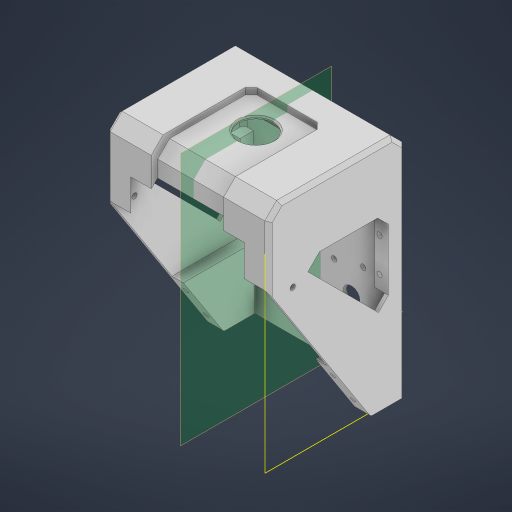
# Autodesk Inventor part: Head_base_mount
Saved by Autodesk Inventor 2024 (Build 280153000, 153)
## iProperties
Created: 2025-09-25
Part Number: Head_base_mount
Material: Generic
Document SubType Name: Modeling
Designer: kevin
Density: 1 g/cm^3
Appearance: Default
Author: kevin
Autodesk Inventor part; units mm, degrees
sketch "Sketch1" plane through (0, 0, 0) normal (0, 0, 1) x (1, 0, 0)
  circle A0 centre (57.1655, 18.417) radius 2.1 projected
  circle A1 centre (12.7885, 12.5269) radius 2.1 projected
  circle A2 centre (17.2869, -26.8107) radius 2.1 projected
  circle A3 centre (-1.1004, -6.0436) radius 5 projected
  line L0 (64.4194, 6.1067) -> (62.3371, -1.6056) projected
  line L1 (67.3095, 9.3686) -> (64.4194, 6.1067) projected
  ellipse E0 centre (57.1655, 18.417) end of major axis (47.0979, 27.5508) minor radius 11.51 (67.3095, 9.3686) -> (68.6853, 21.7358) ccw projected
  ellipse E1 centre (54.4602, 15.4351) end of major axis (43.6731, 3.5452) minor radius 13.5934 (68.6853, 21.7358) -> (59.3507, 30.2045) ccw projected
  ellipse E2 centre (57.1655, 18.417) end of major axis (47.0979, 27.5508) minor radius 11.51 (59.3507, 30.2045) -> (47.0214, 27.4655) ccw projected
  line L2 (36.5043, 15.5956) -> (47.0214, 27.4655) projected
  arc A4 (36.5043, 15.5956) -> (29.6862, 12.4398) centre (33.7853, 12.5269) ccw projected
  line L3 (16.8875, 12.4398) -> (29.6862, 12.4398) projected
  arc A5 (16.8875, 12.4398) -> (10.0695, 15.5956) centre (12.7885, 12.5269) ccw projected
  line L4 (10.0695, 15.5956) -> (-0.4476, 27.4655) projected
  ellipse E3 centre (-10.5917, 18.417) end of major axis (-0.5241, 27.5508) minor radius 11.51 (-0.4476, 27.4655) -> (-12.7769, 30.2045) ccw projected
  ellipse E4 centre (-7.8864, 15.4351) end of major axis (2.9006, 3.5452) minor radius 13.5934 (-12.7769, 30.2045) -> (-22.1115, 21.7358) ccw projected
  ellipse E5 centre (-10.5917, 18.417) end of major axis (-0.5241, 27.5508) minor radius 11.51 (-22.1115, 21.7358) -> (-20.7358, 9.3686) ccw projected
  line L5 (-20.7358, 9.3686) -> (-17.8456, 6.1067) projected
  line L6 (-17.8456, 6.1067) -> (-15.7633, -1.6056) projected
  line L7 (-15.7633, -1.6056) -> (-6.4546, -11.2249) projected
  line L8 (-6.4546, -11.2249) -> (1.9738, -21.6241) projected
  line L9 (1.9738, -21.6241) -> (9.6038, -24.7107) projected
  line L10 (9.6038, -24.7107) -> (14.4693, -29.7892) projected
  arc A6 (14.4693, -29.7892) -> (17.2869, -30.9107) centre (17.2869, -26.8107) ccw projected
  line L11 (17.2869, -30.9107) -> (29.2869, -30.9107) projected
  arc A7 (29.2869, -30.9107) -> (32.1045, -29.7892) centre (29.2869, -26.8107) ccw projected
  line L12 (36.97, -24.7107) -> (32.1045, -29.7892) projected
  line L13 (44.6, -21.6241) -> (36.97, -24.7107) projected
  line L14 (53.0284, -11.2249) -> (44.6, -21.6241) projected
  line L15 (62.3371, -1.6056) -> (53.0284, -11.2249) projected
  circle A8 centre (-10.5917, 18.417) radius 2.1 projected
  circle A9 centre (47.6742, -6.0436) radius 5 projected
  circle A10 centre (29.2869, -26.8107) radius 2.1 projected
  circle A11 centre (33.7853, 12.5269) radius 2.1 projected
  line L16 (23.0369, -57.3492) -> (23.0369, -47.5992) projected
  line L17 (88.0369, 125.5308) -> (-41.9631, 125.5308)
  line L18 (-41.9631, 125.5308) -> (-41.9631, -57.3492)
  line L19 (-41.9631, -57.3492) -> (88.0369, -57.3492)
  line L20 (88.0369, -57.3492) -> (88.0369, 125.5308)
  line L21 (88.0369, 125.5308) -> (-41.9631, -57.3492) construction
  line L22 (-41.9631, 125.5308) -> (88.0369, -57.3492) construction
  circle A12 centre (47.6742, -6.0436) radius 6.75
  circle A13 centre (-1.1004, -6.0436) radius 6.75
  line L23 (33.1369, 106.1308) -> (33.1369, 113.8808) projected
  line L24 (12.9369, 113.8808) -> (12.9369, 106.1308) projected
  line L25 (33.1369, 110.0058) -> (12.9369, 110.0058) construction
  circle A14 centre (34.0369, 59.4461) radius 2.1
  circle A15 centre (23.0369, 69.6441) radius 2.1
  circle A16 centre (12.0369, 59.4461) radius 2.1
  line L26 (23.0369, 12.4398) -> (23.0369, -30.9107) construction
  arc A17 (10.7829, 39.5316) -> (35.2909, 39.5316) centre (23.0369, 31.7099) ccw construction
  line L27 (23.0369, 31.7099) -> (23.0369, -30.9107) construction
  line L28 (23.0369, 31.7099) -> (23.0369, 44.0027) construction
  point P0 (0, 0)
  point P1 (23.0369, 34.0908)
  dimension "d0" = 130
  dimension "d1" = 182.88
  dimension "d2" = 1.75
  dimension "d3" = 1.75
  dimension "d49" = 4.2
  dimension "d51" = 4.2
  dimension "d52" = 15
  constraints: 20 end point, 6 centre point, 4 midpoint, 3 parallel, 2 point on circle, 2 point on line, 2 vertical, 1 horizontal, 1 perpendicular, 10 other
  measures "d0" distance of L19.end L18.end
  measures "d1" distance of L18.end L17.end
  measures "d2" radial gap between concentric circles of A9 A12
  measures "d3" radial gap between concentric circles of A3 A13
  measures "d49" diameter of A14
  measures "d51" diameter of A15
  measures "d52" distance of A15.centre A14.centre
extrude "Extrusion1" add sketch "Sketch1" along normal blind 3 contours L0 L15 L14 L13 L12 A7 L11 A6 L10 L9 L8 L7 L6 L5 E5 E4 E3 L4 A5 L3 A4 L2 E2 E1 E0 L1 | L20 L19 L18 L17
ref_plane "Work Plane1" through (0, 0, 55) normal (0, 0, -1) x (-1, 0, 0)
ref_plane "Work Plane2" through (23.0369, -57.3492, 0) normal (-1, 0, 0) x (0, 0, 1)
ref_plane "Work Plane3" through (-41.9631, 120.0308, 0) normal (0, 1, 0) x (1, 0, 0)
ref_plane "Work Plane5" through (85.0369, 95.5308, 39.1468) normal (0, 0, -1) x (-1, 0, 0)
sketch "Sketch3" plane through (85.0369, 95.5308, 39.1468) normal (0, 0, -1) x (-1, 0, 0)
  line L0 (51.9, 10.6) -> (51.9, 18.35) projected
  line L1 (51.9, 18.35) -> (72.1, 18.35) projected
  line L2 (72.1, 18.35) -> (72.1, 10.6) projected
  line L3 (72.1, 10.6) -> (51.9, 10.6) projected
  line L4 (108.35, 2) -> (15.65, 2) projected
  line L5 (108.35, 22.6942) -> (108.35, 2) projected
  line L6 (87.7096, 24.5) -> (108.35, 22.6942) projected
  line L7 (36.2904, 24.5) -> (87.7096, 24.5) projected
  line L8 (15.65, 22.6942) -> (36.2904, 24.5) projected
  line L9 (15.65, 22.6942) -> (15.65, 2) projected
  line L10 (72.5, 18.75) -> (51.5, 18.75)
  line L11 (51.5, 18.75) -> (51.5, 10.2)
  line L12 (51.5, 10.2) -> (72.5, 10.2)
  line L13 (72.5, 10.2) -> (72.5, 18.75)
  line L14 (51.5, 18.35) -> (39.8, 18.35)
  line L15 (39.8, 18.35) -> (39.8, 10.6)
  line L16 (39.8, 10.6) -> (51.5, 10.6)
  line L17 (62, 18.35) -> (62, 14.8844) construction
  line L18 (39.8, 18.35) -> (15.65, 18.75)
  line L19 (39.8, 10.6) -> (15.65, 11)
  line L20 (72.5, 18.35) -> (84.2, 18.35)
  line L21 (84.2, 18.35) -> (84.2, 10.6)
  line L22 (84.2, 10.6) -> (72.5, 10.6)
  line L23 (84.2, 18.35) -> (108.35, 18.75)
  line L24 (84.2, 10.6) -> (108.35, 11)
  point P0 (85.0369, -95.5308)
  point P1 (108.35, 11)
  point P2 (108.35, 18.75)
  dimension "d8" = 0.4
  dimension "d9" = 11.7
  constraints: 30 end point, 6 symmetric about line, 4 point on line, 2 perpendicular, 1 horizontal, 1 midpoint, 1 parallel, 1 vertical, 3 other
  measures "d8" distance between parallel lines of L1 L10
  measures "d9" distance of L14.start L14.end
extrude "Extrusion2" add sketch "Sketch3" along normal blind 9.398 contours L4 L9 L19 L16 L11 L12 L13 L22 L24 L5 | L23 L20 L13 L10 L11 L14 L18 L9 L8 L7 L6 L5 | L22 L13 L20 L21 | L15 L14 L11 L16
sketch "Sketch4" plane through (0.8369, 106.1308, 39.1468) normal (-1, 0, 0) x (0, 0, 1)
  circle A0 centre (-4.6468, 3.875) radius 2.25 projected
  point P0 (-39.1468, -106.1308)
extrude "Extrusion3" cut sketch "Sketch4" against normal up to surface (44.4 mm away)
sketch "Sketch5" plane through (0.8369, 106.1308, 39.1468) normal (-1, 0, 0) x (0, 0, 1)
  circle A0 centre (-4.6468, 3.875) radius 2.25 projected
  circle A1 centre (-4.6468, 3.875) radius 3.3
  point P0 (-39.1468, -106.1308)
  dimension "d14" = 6.6
  constraints: 1 centre point, 1 coincident
  measures "d14" diameter of A1
extrude "Extrusion4" cut sketch "Sketch5" against normal blind 3.5
sketch "Sketch6" plane through (45.2369, 106.1308, 39.1468) normal (1, 0, 0) x (0, 0, -1)
  circle A0 centre (4.6468, 3.875) radius 2.25 projected
  circle A1 centre (4.6468, 3.875) radius 3.3
  point P0 (39.1468, -106.1308)
  dimension "d17" = 6.6
  constraints: 1 centre point, 1 coincident
  measures "d17" diameter of A1
extrude "Extrusion5" cut sketch "Sketch6" against normal blind 3.5 contours A0 | A1
sketch "Sketch7" plane through (85.0369, 95.5308, 29.7488) normal (0, 0, -1) x (-1, 0, 0)
  line L0 (15.65, 11) -> (15.65, 2) projected
  line L1 (15.65, 2) -> (108.35, 2) projected
  line L2 (108.35, 2) -> (108.35, 11) projected
  line L3 (108.35, 11) -> (84.2, 10.6) projected
  line L4 (84.2, 10.6) -> (84.2, 18.35) projected
  line L5 (84.2, 18.35) -> (108.35, 18.75) projected
  line L6 (108.35, 18.75) -> (108.35, 22.6942) projected
  line L7 (108.35, 22.6942) -> (87.7096, 24.5) projected
  line L8 (87.7096, 24.5) -> (36.2904, 24.5) projected
  line L9 (36.2904, 24.5) -> (15.65, 22.6942) projected
  line L10 (15.65, 22.6942) -> (15.65, 18.75) projected
  line L11 (15.65, 18.75) -> (39.8, 18.35) projected
  line L12 (39.8, 18.35) -> (39.8, 10.6) projected
  line L13 (39.8, 10.6) -> (15.65, 11) projected
  line L14 (51.5, 10.2) -> (51.5, 18.75) projected
  line L15 (51.5, 18.75) -> (72.5, 18.75) projected
  line L16 (72.5, 18.75) -> (72.5, 10.2) projected
  line L17 (72.5, 10.2) -> (51.5, 10.2) projected
  line L18 (15.65, 11) -> (15.65, 18.75)
  line L19 (108.35, 18.75) -> (108.35, 11)
  point P0 (85.0369, -95.5308)
  constraints: 4 end point, 1 parallel, 1 point on line
extrude "Extrusion6" add sketch "Sketch7" along normal up to surface (26.7488 mm away) contours L13 L12 L11 L10 L9 L8 L7 L6 L5 L4 L3 L2 L1 L0 | L18 L11 L12 L13 | L3 L4 L5 L19 | L14 L15 L16 L17
sketch "Sketch8" plane through (0, 0, 3) normal (0, 0, 1) x (1, 0, 0)
  line L0 (69.3869, 97.5308) -> (-23.3131, 97.5308) projected
  line L1 (-23.3131, 97.5308) -> (-23.3131, 118.225) projected
  line L2 (-23.3131, 118.225) -> (-2.6727, 120.0308) projected
  line L3 (-2.6727, 120.0308) -> (48.7465, 120.0308) projected
  line L4 (48.7465, 120.0308) -> (69.3869, 118.225) projected
  line L5 (69.3869, 118.225) -> (69.3869, 97.5308) projected
  line L6 (-41.9631, -57.3492) -> (88.0369, -57.3492) projected
  line L7 (88.0369, -57.3492) -> (88.0369, 125.5308) projected
  line L8 (88.0369, 125.5308) -> (-41.9631, 125.5308) projected
  line L9 (-41.9631, 125.5308) -> (-41.9631, -57.3492) projected
  circle A0 centre (12.7885, 12.5269) radius 2.1 projected
  circle A1 centre (33.7853, 12.5269) radius 2.1 projected
  circle A2 centre (47.6742, -6.0436) radius 6.75 projected
  circle A3 centre (-1.1004, -6.0436) radius 6.75 projected
  circle A4 centre (29.2869, -26.8107) radius 2.1 projected
  circle A5 centre (-10.5917, 18.417) radius 2.1 projected
  circle A6 centre (17.2869, -26.8107) radius 2.1 projected
  circle A7 centre (57.1655, 18.417) radius 2.1 projected
  line L10 (85.0369, 122.5308) -> (85.0369, -57.3492)
  line L11 (85.0369, -54.3492) -> (-38.9631, -54.3492) construction
  line L12 (-38.9631, -57.3492) -> (-38.9631, 122.5308)
  line L13 (-38.9631, 122.5308) -> (85.0369, 122.5308) construction
  line L14 (-23.3131, 114.2808) -> (-38.9631, 114.2808)
  line L15 (23.0369, -93.9252) -> (23.0369, 162.1068) construction
  line L16 (69.3869, 114.2808) -> (85.0369, 114.2808)
  line L17 (85.0369, -52.3492) -> (-38.9631, -52.3492) construction
  point P0 (0, 0)
  dimension "d23" = 3
  dimension "d24" = 2
  constraints: 14 end point, 5 point on line, 2 symmetric about line, 1 parallel, 1 perpendicular
  measures "d23" distance between parallel lines of L7 L10
  measures "d24" distance between parallel lines of L11 L17
extrude "Extrusion7" add sketch "Sketch8" along normal blind 27 contours L5 L4 L3 L2 L1 L14 L12 L6 L9 L8 L7 L10 L16
sketch "Sketch9" plane through (0, 0, 30) normal (0, 0, 1) x (1, 0, 0)
  line L0 (69.3869, 114.2808) -> (69.3869, 118.225) projected
  line L1 (69.3869, 114.2808) -> (85.0369, 114.2808) projected
  line L2 (85.0369, 114.2808) -> (85.0369, -57.3492) projected
  line L3 (85.0369, -57.3492) -> (88.0369, -57.3492) projected
  line L4 (88.0369, -57.3492) -> (88.0369, 125.5308) projected
  line L5 (88.0369, 125.5308) -> (-41.9631, 125.5308) projected
  line L6 (-41.9631, 125.5308) -> (-41.9631, -57.3492) projected
  line L7 (-41.9631, -57.3492) -> (-38.9631, -57.3492) projected
  line L8 (-38.9631, -57.3492) -> (-38.9631, 114.2808) projected
  line L9 (-38.9631, 114.2808) -> (-23.3131, 114.2808) projected
  line L10 (-23.3131, 118.225) -> (-23.3131, 114.2808) projected
  line L11 (-2.6727, 120.0308) -> (-23.3131, 118.225) projected
  line L12 (48.7465, 120.0308) -> (-2.6727, 120.0308) projected
  line L13 (69.3869, 118.225) -> (48.7465, 120.0308) projected
  line L14 (-2.6945, 120.5308) -> (-23.8131, 118.6832) construction
  line L15 (-39.4631, -56.8492) -> (-41.4631, -56.8492)
  line L16 (87.5369, -56.8492) -> (85.5369, -56.8492)
  line L17 (69.8869, 118.6832) -> (48.7683, 120.5308) construction
  line L18 (52.0369, 120.5308) -> (-5.9631, 120.5308)
  line L19 (-2.7818, 122.5308) -> (52.0369, 122.5308)
  line L20 (88.0369, 125.5308) -> (-41.9631, 125.5308) projected
  line L21 (52.0369, 125.5308) -> (52.0369, 106.9413)
  line L22 (58.0369, 122.5308) -> (-5.9631, 122.5308)
  line L23 (23.0369, 125.5308) -> (23.0369, 133.2517) construction
  line L24 (-5.9631, 125.5308) -> (-5.9631, 106.9413)
  line L25 (88.0369, 120.5308) -> (52.0369, 120.5308)
  line L26 (-5.9631, 120.5308) -> (-41.9631, 120.5308)
  line L27 (-41.9631, 116.0058) -> (-41.9631, 125.5308) projected
  line L28 (-38.9631, 114.2808) -> (-38.9631, 120.5308)
  line L29 (85.0369, 114.2808) -> (85.0369, 120.5308)
  point P0 (0, 0)
  point P1 (52.0369, 120.2449)
  point P2 (26.13, 122.5308)
  point P3 (-5.9631, 125.5308)
  dimension "d30" = 0.5
  dimension "d31" = 2
  dimension "d32" = 36
  dimension "d38" = 5
  dimension "d40" = 5
  constraints: 28 end point, 13 point on line, 4 perpendicular, 2 symmetric about line, 2 vertical, 1 midpoint
  measures "d30" distance between parallel lines of L12 L18
  measures "d31" distance between parallel lines of L18 L19
  measures "d32" distance between parallel lines of L4 L21
  measures "d38" distance between parallel lines of L5 L25
  measures "d40" distance between parallel lines of L5 L26
ref_plane "Work Plane6" through (23.0369, 120.0308, 55) normal (0, 1, 0) x (-1, 0, 0)
sketch "Sketch10" plane through (23.0369, 120.0308, 55) normal (0, 1, 0) x (-1, 0, 0)
  circle A0 centre (0, 0) radius 11.975 projected
  circle A1 centre (0, 0) radius 7.8185 projected
  circle A2 centre (0, 0) radius 13.975
  point P0 (23.0369, -55)
  dimension "d33" = 2
  constraints: 1 centre point
  measures "d33" radial gap between concentric circles of A0 A2
extrude "Extrusion8" add sketch "Sketch9" along normal blind 80 contours L29 L25 L4 L3 L2 | L25 L21 L5 L4 | L18 L24 L22 L19 L21 | L26 L6 L5 L24 | L28 L8 L7 L6 L26
extrude "Extrusion9" cut sketch "Sketch10" along normal blind 80 contours A0 | A1 | A2
sketch "Sketch11" plane through (-41.9631, 125.5308, 0) normal (0, 1, 0) x (1, 0, 0)
  line L0 (130, 0) -> (0, 0) projected
  line L1 (0, 0) -> (0, -110) projected
  line L2 (36, -110) -> (0, -110) projected
  line L3 (36, -30) -> (36, -110) projected
  line L4 (94, -30) -> (36, -30) projected
  line L5 (94, -30) -> (94, -110) projected
  line L6 (130, -110) -> (94, -110) projected
  line L7 (130, 0) -> (130, -110) projected
  point P0 (41.9631, 0)
extrude "Extrusion10" add sketch "Sketch11" along normal blind 2
sketch "Sketch12" plane through (85.0369, -57.3492, 3) normal (-1, 0, 0) x (0, 0, 1)
  line L0 (0, 0) -> (0, 171.63) projected
  line L1 (0, 0) -> (107, 0) projected
  line L2 (107, 177.88) -> (107, 0) projected
  line L3 (27, 177.88) -> (107, 177.88) projected
  line L4 (27, 171.63) -> (27, 177.88) projected
  line L5 (0, 171.63) -> (27, 171.63) projected
  line L6 (107, 152.1906) -> (81.3106, 177.88)
  line L7 (67.65, 175.5742) -> (67.65, 154.88) construction
  point P0 (-3, 57.3492)
  dimension "d43" = 45
  constraints: 2 end point, 2 point on line
  measures "d43" angle of L2 L6
extrude "Extrusion11" add sketch "Sketch12" along normal up to surface (124 mm away) contours L6 L3 L2
sketch "Sketch13" plane through (0, 0, 110) normal (0, 0, 1) x (1, 0, 0)
  line L0 (85.0369, 94.8414) -> (-38.9631, 94.8414) projected
  line L1 (85.0369, 94.8414) -> (85.0369, -57.3492) projected
  line L2 (85.0369, -57.3492) -> (88.0369, -57.3492) projected
  line L3 (88.0369, -57.3492) -> (88.0369, 127.5308) projected
  line L4 (52.0369, 127.5308) -> (88.0369, 127.5308) projected
  line L5 (52.0369, 122.5308) -> (52.0369, 127.5308) projected
  line L6 (52.0369, 122.5308) -> (-5.9631, 122.5308) projected
  line L7 (-5.9631, 122.5308) -> (-5.9631, 127.5308) projected
  line L8 (-41.9631, 127.5308) -> (-5.9631, 127.5308) projected
  line L9 (-41.9631, -57.3492) -> (-41.9631, 127.5308) projected
  line L10 (-41.9631, -57.3492) -> (-38.9631, -57.3492) projected
  line L11 (-38.9631, -57.3492) -> (-38.9631, 94.8414) projected
  line L12 (52.0369, 128.7536) -> (52.0369, 94.8414)
  line L13 (-5.9631, 127.5308) -> (-5.9631, 94.8414)
  point P0 (0, 0)
  constraints: 4 end point, 2 perpendicular, 2 point on line
extrude "Extrusion12" cut sketch "Sketch13" against normal blind 5 contours L0 L13 L6 L12
fillet "Fillet2" radius 1 3 edges at (14.317, 122.5308, 65.9208) (14.317, 122.5308, 44.0792) (37.0119, 122.5308, 55) inverted yes
sketch "Sketch14" plane through (85.0369, -57.3492, 3) normal (-1, 0, 0) x (0, 0, 1)
  line L0 (107, 152.1906) -> (81.3106, 177.88) projected
  line L1 (27, 177.88) -> (81.3106, 177.88) projected
  line L2 (27, 171.63) -> (27, 177.88) projected
  line L3 (0, 171.63) -> (27, 171.63) projected
  line L4 (0, 0) -> (0, 171.63) projected
  line L5 (0, 0) -> (107, 0) projected
  line L6 (107, 152.1906) -> (107, 0) projected
  point P0 (-3, 57.3492)
sketch "Sketch15" plane through (85.0369, -57.3492, 3) normal (-1, 0, 0) x (0, 0, 1)
  line L0 (107, 152.1906) -> (81.3106, 177.88) projected
  line L1 (27, 177.88) -> (81.3106, 177.88) projected
  line L2 (27, 171.63) -> (27, 177.88) projected
  line L3 (0, 171.63) -> (27, 171.63) projected
  line L4 (0, 0) -> (0, 171.63) projected
  line L5 (0, 0) -> (107, 0) projected
  line L6 (107, 152.1906) -> (107, 0) projected
  line L7 (25, 0) -> (107, 127)
  point P0 (-3, 57.3492)
  dimension "d56" = 25
  dimension "d57" = 127
  constraints: 2 end point, 2 point on line
  measures "d56" distance of L4.start L7.start
  measures "d57" distance of L5.end L7.end
extrude "Extrusion13" cut sketch "Sketch15" along normal blind 225.25 and the other way blind 7.8486 contours L6 L5 L7
ref_plane "Work Plane7" through (54.0369, 69.6508, 110) normal (0, -1, 0) x (1, 0, 0)
sketch "Sketch19" plane through (85.0369, 95.5308, 39.1468) normal (0, 0, 1) x (1, 0, 0)
  line L0 (-51.9, 10.6) -> (-51.9, 18.35) projected
  line L1 (-51.9, 18.35) -> (-72.1, 18.35) projected
  line L2 (-72.1, 18.35) -> (-72.1, 10.6) projected
  line L3 (-72.1, 10.6) -> (-51.9, 10.6) projected
  line L4 (-108.35, 2) -> (-15.65, 2) projected
  line L5 (-108.35, 22.6942) -> (-108.35, 2) projected
  line L6 (-87.7096, 24.5) -> (-108.35, 22.6942) projected
  line L7 (-36.2904, 24.5) -> (-87.7096, 24.5) projected
  line L8 (-15.65, 22.6942) -> (-36.2904, 24.5) projected
  line L9 (-15.65, 22.6942) -> (-15.65, 2) projected
  line L10 (-108.55, 1.8) -> (-15.45, 1.8)
  line L11 (-15.45, 1.8) -> (-15.45, 22.8775)
  line L12 (-15.45, 22.8775) -> (-36.2817, 24.7)
  line L13 (-36.2817, 24.7) -> (-87.7183, 24.7)
  line L14 (-87.7183, 24.7) -> (-108.55, 22.8775)
  line L15 (-108.55, 22.8775) -> (-108.55, 1.8)
  point P0 (-85.0369, -95.5308)
  dimension "d71" = 0.2
  constraints: 12 end point, 5 other
  measures "d71" distance between parallel lines of L5 L15
extrude "Extrusion16" cut sketch "Sketch19" against normal blind 19.498 contours L3 L2 L1 L0 | L5 L6 L7 L8 L9 L4 | L15 L14 L13 L12 L11 L10
ref_plane "Work Plane9" through (23.0369, -57.3492, 0) normal (-1, 0, 0) x (0, 0, 1)
sketch "Sketch21" plane through (0, 0, 0) normal (0, 0, -1) x (-1, 0, 0)
  line L0 (23.3131, 114.2808) -> (23.5131, 114.2808) projected
  line L1 (23.3131, 97.5308) -> (23.3131, 114.2808) projected
  line L2 (-69.3869, 97.5308) -> (23.3131, 97.5308) projected
  line L3 (-69.3869, 114.2808) -> (-69.3869, 97.5308) projected
  line L4 (-69.5869, 114.2808) -> (-69.3869, 114.2808) projected
  line L5 (-69.5869, 118.4083) -> (-69.5869, 114.2808) projected
  line L6 (-48.7552, 120.2308) -> (-69.5869, 118.4083) projected
  line L7 (2.6814, 120.2308) -> (-48.7552, 120.2308) projected
  line L8 (23.5131, 118.4083) -> (2.6814, 120.2308) projected
  line L9 (23.5131, 114.2808) -> (23.5131, 118.4083) projected
  circle A0 centre (11.3131, 107.8779) radius 2.1 projected
  circle A1 centre (-23.3827, 107.8779) radius 2.1 projected
  circle A2 centre (-58.0785, 107.8779) radius 2.1 projected
  point P0 (0, 0)
ref_plane "Work Plane10" through (-23.3131, 97.5308, 19.6488) normal (0, 0, -1) x (0, 1, 0)
extrude "Extrusion17" cut sketch "Sketch21" against normal up to surface (19.6488 mm away) contours A0 | A1 | A2
sketch "Sketch22" plane through (0, 0, 0) normal (0, 0, -1) x (-1, 0, 0)
  circle A0 centre (-58.0785, 107.8779) radius 2.1 projected
  circle A1 centre (11.3131, 107.8779) radius 2.1 projected
  circle A2 centre (-23.3827, 107.8779) radius 2.1 projected
  line L0 (-88.0369, -57.3492) -> (-88.0369, 127.5308) projected
  line L1 (41.9631, -57.3492) -> (-88.0369, -57.3492) projected
  line L2 (41.9631, -57.3492) -> (41.9631, 127.5308) projected
  circle A3 centre (-23.0369, 69.6441) radius 2.1 projected
  circle A4 centre (-34.0369, 59.4461) radius 2.1 projected
  circle A5 centre (-12.0369, 59.4461) radius 2.1 projected
  circle A6 centre (-29.2869, -26.8107) radius 2.1 projected
  circle A7 centre (10.5917, 18.417) radius 2.1 projected
  circle A8 centre (-17.2869, -26.8107) radius 2.1 projected
  circle A9 centre (-57.1655, 18.417) radius 2.1 projected
  circle A10 centre (1.1004, -6.0436) radius 6.75 projected
  circle A11 centre (-47.6742, -6.0436) radius 6.75 projected
  circle A12 centre (-33.7853, 12.5269) radius 2.1 projected
  circle A13 centre (-12.7885, 12.5269) radius 2.1 projected
  circle A14 centre (11.3131, 107.8779) radius 4
  circle A15 centre (-23.3827, 107.8779) radius 4
  circle A16 centre (-58.0785, 107.8779) radius 4
  line L3 (-88.0369, 127.5308) -> (41.9631, 127.5308) projected
  point P0 (0, 0)
  dimension "d76" = 8
  dimension "d77" = 8
  dimension "d78" = 8
  constraints: 3 centre point, 3 coincident
  measures "d76" diameter of A14
  measures "d77" diameter of A15
  measures "d78" diameter of A16
extrude "Extrusion18" cut sketch "Sketch22" against normal blind 3 contours A14 | A15 | A16
chamfer "Chamfer3" distance 9.525 angle 45 4 edges at (23.0369, 127.5308, 0) (-23.9631, 127.5308, 110) (23.0369, 122.5308, 105) (70.0369, 127.5308, 110)
sketch "Sketch23" plane through (-41.9631, 127.5308, 0) normal (0, 1, 0) x (1, 0, 0)
  line L0 (130, -100.475) -> (94, -100.475) projected
  line L1 (130, -100.475) -> (130, -9.525) projected
  line L2 (0, -9.525) -> (130, -9.525) projected
  line L3 (0, -9.525) -> (0, -100.475) projected
  line L4 (36, -100.475) -> (0, -100.475) projected
  line L5 (36, -100.475) -> (36, -30) projected
  line L6 (36, -30) -> (94, -30) projected
  line L7 (94, -30) -> (94, -100.475) projected
  line L8 (94, -34.8149) -> (89.1851, -30)
  line L9 (65, -30) -> (65, -25.0222) construction
  line L10 (36, -34.8149) -> (40.8149, -30)
  point P0 (41.9631, 0)
  dimension "d84" = 45
  constraints: 6 end point, 2 point on line, 2 symmetric about line, 1 midpoint, 1 vertical
  measures "d84" angle of L6 L8
extrude "Extrusion19" add sketch "Sketch23" against normal up to surface (5 mm away) contours L8 L6 L7 | L10 L5 L6
sketch "Sketch25" plane through (85.0369, -57.3492, 3) normal (-1, 0, 0) x (0, 0, 1)
  line L0 (25, 0) -> (107, 127) projected
  line L1 (107, 152.1906) -> (107, 127) projected
  line L2 (107, 152.1906) -> (81.3106, 177.88) projected
  line L3 (27, 177.88) -> (81.3106, 177.88) projected
  line L4 (27, 171.63) -> (27, 177.88) projected
  line L5 (0, 171.63) -> (27, 171.63) projected
  line L6 (0, 0) -> (0, 171.63) projected
  line L7 (0, 0) -> (25, 0) projected
  line L8 (0, 0) -> (0, 171.63) projected
  line L9 (0, 50) -> (57.2835, 50)
  line L10 (25, 0) -> (107, 127) projected
  point P0 (-3, 57.3492)
  dimension "d87" = 50
  constraints: 2 end point, 2 point on line, 1 horizontal
  measures "d87" distance between parallel lines of L7 L9
extrude "Extrusion20" add sketch "Sketch25" along normal blind 9 contours L7 L6 L9 L0
mirror "Mirror1" about plane through (23.0369, -57.3492, 0) normal (-1, 0, 0) of "Extrusion20"
sketch "Sketch26" plane through (-41.9631, -57.3492, 0) normal (0, -1, 0) x (1, 0, 0)
  line L0 (0, 28) -> (12, 28) projected
  line L1 (0, 0) -> (0, 28) projected
  line L2 (0, 0) -> (130, 0) projected
  line L3 (130, 0) -> (130, 28) projected
  line L4 (130, 28) -> (118, 28) projected
  line L5 (118, 3) -> (118, 28) projected
  line L6 (12, 3) -> (118, 3) projected
  line L7 (12, 3) -> (12, 28) projected
  line L8 (12, 3) -> (0, 3)
  line L9 (118, 3) -> (118, 28) projected
  line L10 (118, 3) -> (130, 3)
  line L11 (124, 3) -> (124, 28) construction
  line L12 (6, 3) -> (6, 28) construction
  circle A0 centre (6, 11) radius 2.1
  line L13 (65, 0) -> (65, 3) construction
  circle A1 centre (124, 11) radius 2.1
  point P0 (41.9631, 0)
  dimension "d90" = 4.2
  dimension "d91" = 8
  constraints: 10 end point, 6 midpoint, 4 point on line, 2 centre point, 1 perpendicular, 1 symmetric about line, 1 other
  measures "d90" diameter of A0
  measures "d91" distance from line of L8 A0.centre
extrude "Extrusion21" cut sketch "Sketch26" against normal blind 9 contours A0 | A1
sketch "Sketch27" plane through (-41.9631, -57.3492, 28) normal (0, -0.5424282, 0.8401022) x (1, 0, 0)
  line L0 (3, 151.1721) -> (3, 59.5166) projected
  line L1 (0, 151.1721) -> (3, 151.1721) projected
  line L2 (0, 0) -> (0, 151.1721) projected
  line L3 (0, 0) -> (12, 0) projected
  line L4 (12, 0) -> (12, 59.5166) projected
  line L5 (3, 59.5166) -> (12, 59.5166) projected
  line L6 (130, 151.1721) -> (130, 0) projected
  line L7 (127, 151.1721) -> (130, 151.1721) projected
  line L8 (127, 59.5166) -> (127, 151.1721) projected
  line L9 (127, 59.5166) -> (118, 59.5166) projected
  line L10 (118, 0) -> (118, 59.5166) projected
  line L11 (130, 0) -> (118, 0) projected
  circle A0 centre (6, 44.5166) radius 2.1
  circle A1 centre (6, 15) radius 2.1
  line L12 (12, 0) -> (118, 0) construction
  line L13 (65, 0) -> (65, 18.5988) construction
  line L14 (6, 0) -> (6, 59.5166) construction
  circle A2 centre (124, 44.5166) radius 2.1
  circle A3 centre (124, 15) radius 2.1
  point P0 (41.9631, 32.9912)
  dimension "d94" = 4.2
  dimension "d95" = 4.2
  dimension "d96" = 15
  dimension "d97" = 15
  constraints: 6 end point, 4 centre point, 3 point on line, 2 midpoint, 2 symmetric about line, 1 horizontal, 1 perpendicular, 1 vertical, 2 other
  measures "d94" diameter of A0
  measures "d95" diameter of A1
  measures "d96" distance from line of L5 A0.centre
  measures "d97" distance from line of L3 A1.centre
extrude "Extrusion22" cut sketch "Sketch27" against normal blind 9 contours A0 | A1 | A2 | A3
sketch "Sketch28" plane through (-41.9631, -57.3492, 0) normal (-1, 0, 0) x (0, 0, 1)
  line L0 (100.475, 184.88) -> (110, 175.355) projected
  line L1 (9.525, 184.88) -> (100.475, 184.88) projected
  line L2 (0, 175.355) -> (9.525, 184.88) projected
  line L3 (0, 0) -> (0, 175.355) projected
  line L4 (0, 0) -> (28, 0) projected
  line L5 (28, 0) -> (110, 127) projected
  line L6 (110, 127) -> (110, 175.355) projected
  line L7 (13.8224, 135.0021) -> (13.8224, 61.0664)
  line L8 (13.8224, 61.0664) -> (87.7581, 135.0021)
  line L9 (13.8224, 135.0021) -> (101.5696, 135.0021)
  line L10 (60.2835, 50) -> (3, 50) construction
  line L11 (22.3653, 135.0021) -> (13.8224, 126.4592)
  line L12 (69, 135.0021) -> (85.8906, 118.1114)
  line L13 (13.8224, 77.0979) -> (26.1283, 64.792)
  point P0 (0, 57.3492)
  point P1 (6, 50)
  point P2 (21.8381, 69.0821)
  point P3 (78.379, 125.623)
  dimension "d101" = 45
  dimension "d104" = 45
  dimension "d105" = 45
  constraints: 12 end point, 5 point on line, 1 horizontal, 1 parallel, 1 perpendicular, 1 vertical
  measures "d101" angle of L7 L8
  measures "d104" angle of L9 L12
  measures "d105" angle of L7 L13
extrude "Extrusion23" cut sketch "Sketch28" against normal up to surface (130 mm away) contours L11 L9 L12 L8 L13 L7
sketch "Sketch29" plane through (0, 0, 3) normal (0, 0, 1) x (1, 0, 0)
  circle A0 centre (12.7885, 12.5269) radius 2.1 projected
  circle A1 centre (33.7853, 12.5269) radius 2.1 projected
  circle A2 centre (47.6742, -6.0436) radius 6.75 projected
  circle A3 centre (-1.1004, -6.0436) radius 6.75 projected
  circle A4 centre (57.1655, 18.417) radius 2.1 projected
  circle A5 centre (17.2869, -26.8107) radius 2.1 projected
  circle A6 centre (-10.5917, 18.417) radius 2.1 projected
  circle A7 centre (29.2869, -26.8107) radius 2.1 projected
  circle A8 centre (12.0369, 59.4461) radius 2.1 projected
  circle A9 centre (34.0369, 59.4461) radius 2.1 projected
  circle A10 centre (23.0369, 69.6441) radius 2.1 projected
  line L0 (-38.9631, -7.3492) -> (-29.9631, -7.3492) projected
  line L1 (-29.9631, -7.3492) -> (-29.9631, -57.3492) projected
  line L2 (-29.9631, -57.3492) -> (76.0369, -57.3492) projected
  line L3 (76.0369, -57.3492) -> (76.0369, -7.3492) projected
  line L4 (76.0369, -7.3492) -> (85.0369, -7.3492) projected
  line L5 (85.0369, -7.3492) -> (85.0369, 114.2808) projected
  line L6 (85.0369, 114.2808) -> (69.3869, 114.2808) projected
  line L7 (69.3869, 114.2808) -> (69.3869, 97.5308) projected
  line L8 (69.3869, 97.5308) -> (-23.3131, 97.5308) projected
  line L9 (-23.3131, 97.5308) -> (-23.3131, 114.2808) projected
  line L10 (-23.3131, 114.2808) -> (-38.9631, 114.2808) projected
  line L11 (-38.9631, 114.2808) -> (-38.9631, -7.3492) projected
  line L12 (-38.9631, 69.11) -> (-38.9631, 19.7487) projected
  line L13 (-38.9631, 69.11) -> (-30.9631, 69.11)
  line L14 (-30.9631, 69.11) -> (-30.9631, 19.7487)
  line L15 (-30.9631, 19.7487) -> (-38.9631, 19.7487)
  line L16 (-38.9631, 19.7487) -> (-38.9631, 69.11)
  line L17 (-34.9631, 69.11) -> (-34.9631, 19.7487) construction
  circle A11 centre (-34.9631, 58.11) radius 2.1
  circle A12 centre (-34.9631, 30.7487) radius 2.1
  point P0 (0, 0)
  dimension "d106" = 8
  dimension "d109" = 4.2
  dimension "d110" = 4.2
  dimension "d111" = 11
  dimension "d112" = 11
  constraints: 10 end point, 3 point on line, 2 centre point, 2 midpoint, 2 parallel, 1 horizontal, 1 perpendicular
  measures "d106" distance of L14.end L15.end
  measures "d109" diameter of A11
  measures "d110" diameter of A12
  measures "d111" distance from line of L13 A11.centre
  measures "d112" distance from line of A12.centre L15
extrude "Extrusion24" add sketch "Sketch29" along normal up to surface (10.8224 mm away) contours L11 L13 L14 L15
mirror "Mirror2" about plane through (23.0369, -57.3492, 0) normal (-1, 0, 0) of "Extrusion24"
sketch "Sketch30" plane through (-41.9631, -57.3492, 0) normal (-1, 0, 0) x (0, 0, 1)
  line L0 (13.8224, 77.0979) -> (13.8224, 126.4592) projected
  line L1 (13.8224, 126.4592) -> (22.3653, 135.0021) projected
  line L2 (22.3653, 135.0021) -> (69, 135.0021) projected
  line L3 (69, 135.0021) -> (78.379, 125.623) projected
  line L4 (78.379, 125.623) -> (21.8381, 69.0821) projected
  line L5 (21.8381, 69.0821) -> (13.8224, 77.0979) projected
  line L6 (100.475, 184.88) -> (110, 175.355) projected
  line L7 (9.525, 184.88) -> (100.475, 184.88) projected
  line L8 (0, 175.355) -> (9.525, 184.88) projected
  line L9 (0, 0) -> (0, 175.355) projected
  line L10 (0, 0) -> (28, 0) projected
  line L11 (28, 0) -> (110, 127) projected
  line L12 (110, 127) -> (110, 175.355) projected
  circle A0 centre (90.5184, 121.032) radius 2.1
  point P0 (0, 57.3492)
  dimension "d113" = 4.2
  constraints: 1 centre point
  measures "d113" diameter of A0
extrude "Extrusion25" cut sketch "Sketch30" against normal up to surface (130 mm away) contours A0
fillet "Fillet4" radius 3 6 edges at (-35.9631, -57.3492, 28) (82.0369, -57.3492, 28) (85.0369, 6.1998, 3) (85.0369, 91.6954, 3) (-38.9631, 91.6954, 3) (-38.9631, 6.1998, 3)
chamfer "Chamfer4" distance 3 angle 45 10 edges at (88.0369, 127.5308, 55) (88.0369, 122.7683, 4.7625) (-41.9631, 122.7683, 4.7625) (-41.9631, 127.5308, 55) (-41.9631, 122.7683, 105.2375) (88.0369, 122.7683, 105.2375) (88.0369, 93.8283, 110) (-41.9631, 93.8283, 110) (-41.9631, 30.3283, 0) (88.0369, 30.3283, 0)
sketch "Sketch31" plane through (54.0369, 69.6508, 110) normal (0, -1, 0) x (1, 0, 0)
  line L0 (-2, 0) -> (-2, -5) projected
  line L1 (-2, -5) -> (-60, -5) projected
  line L2 (-60, -5) -> (-60, 0) projected
  line L3 (-60, 0) -> (-93, 0) projected
  line L4 (-93, -25.6894) -> (-93, 0) projected
  line L5 (31, -25.6894) -> (-93, -25.6894) projected
  line L6 (31, 0) -> (31, -25.6894) projected
  line L7 (31, 0) -> (-2, 0) projected
  line L8 (-93, 0) -> (-93, -49.7165) projected
  line L9 (31, -49.7165) -> (31, 0) projected
  line L10 (-93, -16.5) -> (-76.5, 0)
  line L11 (-31, -5) -> (-31, -11.0894) construction
  line L12 (31, -16.5) -> (14.5, 0)
  point P0 (-54.0369, -110)
  point P1 (31, -16.5)
  point P2 (-93, -16.5)
  dimension "d120" = 45
  constraints: 6 end point, 2 midpoint, 2 symmetric about line, 1 point on line, 1 vertical
  measures "d120" angle of L4 L10
extrude "Extrusion26" add sketch "Sketch31" against normal up to surface contours L7 L6 L12 | L10 L4 L3 surface through (85.0369, 120.5308, 84.3106) normal (0, -0.7071068, -0.7071068)
sketch "Sketch32" plane through (85.0369, 114.2808, 30) normal (-1, 0, 0) x (0, 0, 1)
  line L0 (63.5, -44.63) -> (63.5, -2.9394) projected
  line L1 (63.5, -2.9394) -> (54.3106, 6.25) projected
  line L2 (0, 6.25) -> (54.3106, 6.25) projected
  line L3 (0, 0) -> (0, 6.25) projected
  line L4 (-24, 0) -> (0, 0) projected
  line L5 (-24, -45.1708) -> (-24, 0) projected
  line L6 (-24, -45.1708) -> (-16.1776, -45.1708) projected
  line L7 (-16.1776, -45.1708) -> (-7.6347, -36.6279) projected
  line L8 (-7.6347, -36.6279) -> (39, -36.6279) projected
  line L9 (39, -36.6279) -> (48.379, -46.007) projected
  line L10 (48.379, -46.007) -> (-8.1619, -102.5479) projected
  line L11 (-8.1619, -102.5479) -> (-16.1776, -94.5321) projected
  line L12 (-16.1776, -94.5321) -> (-24, -94.5321) projected
  line L13 (-24, -121.63) -> (-24, -94.5321) projected
  line L14 (-24, -121.63) -> (30.2835, -121.63) projected
  line L15 (30.2835, -121.63) -> (80, -44.63) projected
  line L16 (80, -44.63) -> (63.5, -44.63) projected
  circle A0 centre (60.5184, -50.598) radius 2.1 projected
  line L17 (80, 3.725) -> (80, -44.63) projected
  line L18 (80, -44.63) -> (63.5, -28.13)
  point P0 (-30, -114.2808)
  dimension "d123" = 45
  constraints: 2 end point, 1 point on line
  measures "d123" angle of L0 L18
extrude "Extrusion27" cut sketch "Sketch32" along normal up to surface (124 mm away) contours L0 L18 L16
equation "\"d2\" = d3"
equation "\"d97\" = d96"
equation "\"d110\" = d109"
equation "\"d112\" = d111"
body "Solid1"
